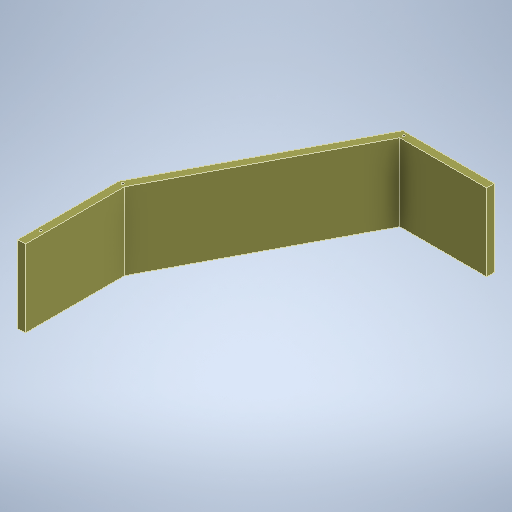
# Autodesk Inventor part: 右仕切り
Saved by Autodesk Inventor 2026.2 (Build 302298010, 298A)
## iProperties
Created: 2026-05-20
Part Number: 右仕切り
Material: 一般
Document SubType Name: Modeling
Designer: Yagis
Density: 1 g/cm^3
Appearance: 既定
Author: Yagis
Autodesk Inventor part; units mm, degrees
ref_plane "YZ Plane" through (0, 0, 0) normal (1, 0, 0) x (0, 1, 0)
ref_plane "XZ Plane" through (0, 0, 0) normal (0, 1, 0) x (-1, 0, 0)
ref_plane "XY Plane" through (0, 0, 0) normal (0, 0, 1) x (1, 0, 0)
sketch "スケッチ1" plane through (0, 0, 0) normal (0, 1, 0) x (-1, 0, 0)
  line L0 (0, 0) -> (8, 0)
  line L1 (8, 0) -> (8, -90)
  line L2 (8, -90) -> (0, -90)
  line L3 (0, -90) -> (0, 0)
  line L4 (-94, -275) -> (-189, -275)
  line L5 (-189, -275) -> (-189, -283)
  line L6 (-189, -283) -> (-94, -283)
  line L7 (-94, -283) -> (-94, -275)
  line L8 (8, -90) -> (-94, -283)
  line L9 (0, -88.016) -> (-98.8205, -275)
  line L10 (8, 0) -> (0, 0)
  line L11 (0, 0) -> (0, 15)
  line L12 (0, 15) -> (8, 15)
  line L13 (8, 15) -> (8, 0)
  dimension "d0" = 8
  dimension "d1" = 90
  dimension "d4" = 8
  dimension "d5" = 185
  dimension "d6" = 94
  dimension "d7" = 8
  dimension "d20" = 95
  dimension "d21" = 15
  constraints: 28 end point, 6 parallel, 3 horizontal, 3 perpendicular, 2 point on line
  measures "d0" distance of L1.end L2.end
  measures "d1" distance of L0.end L1.end
  measures "d4" distance of L4.end L5.end
  measures "d5" distance between parallel lines of L2 L4
  measures "d6" distance between parallel lines of L7 L3
  measures "d7" distance between parallel lines of L9 L8
  measures "d20" distance of L5.end L6.end
  measures "d21" distance of L10.end L11.end
extrude "押し出し1" add sketch "スケッチ1" along normal blind 80
sketch "スケッチ2" plane through (0, 80, 0) normal (0, 1, 0) x (1, 0, 0)
  line L0 (0, -15) -> (0, 88.016) projected
  point P0 (-4, 5)
  point P1 (-4, 90)
  point P2 (99, 279)
  point P3 (-4, 0)
  dimension "d8" = 5
  dimension "d9" = 85
  dimension "d11" = 189
  dimension "d12" = 103
  dimension "d22" = 4
  constraints: 1 vertical alignment
  measures "d8" distance of point (-4, 5) point (-4, 0)
  measures "d9" distance of point (-4, 90) point (-4, 5)
  measures "d11" vertical distance of point (99, 279) point (-4, 90)
  measures "d12" horizontal distance of point (99, 279) point (-4, 90)
  measures "d22" distance from line of L0 point (-4, 5)
hole "穴1" at (-4, 80, -5) at (-4, 80, -90) at (99, 80, -279) direction (0, -1, 0) diameter 2.459 depth 8.8 tip angle 118 thread size "M3x0.5" class "6H" standard "ISO Metric profile"
